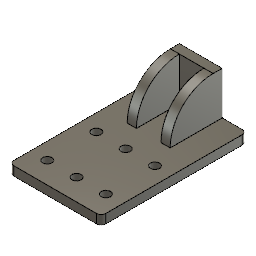
Small_solenoid_basereworkedV1 (Autodesk Fusion 360 design; units mm, degrees)
Autodesk Fusion 360 part; units mm, degrees
note: some values were not read from the file. Set by a fixed rule: which sketch regions a step uses.
sketch "Sketch1" plane through (0, 0, 0) normal (0, 1, 0) x (1, 0, 0)
  line L0 (-15, 15.25) -> (15, 15.25)
  line L1 (15, 15.25) -> (15, -15.25)
  line L2 (15, -15.25) -> (-15, -15.25)
  line L3 (-15, -15.25) -> (-15, 15.25)
  line L4 (-15, 15.25) -> (15, -15.25) construction
  line L5 (15, 15.25) -> (-15, -15.25) construction
  dimension "d1" = 30.5
  dimension "d2" = 30
extrude "Extrude1" add sketch "Sketch1" along normal blind 3
sketch "Sketch2" plane through (0, 0, -15.25) normal (0, 0, -1) x (-1, 0, 0)
  line L0 (-15, 0) -> (15, 0)
  line L1 (15, 0) -> (15, 3)
  line L2 (15, 3) -> (-15, 3)
  line L3 (-15, 3) -> (-15, 0)
  line L4 (7, 0) -> (-7, 0)
  line L5 (-7, 0) -> (-7, 17)
  line L6 (-7, 17) -> (7, 17)
  line L7 (7, 17) -> (7, 0)
  line L8 (7, 1.5) -> (15, 1.5) construction
  line L9 (-15, 1.5) -> (-7, 1.5) construction
  dimension "d5" = 14
  dimension "d6" = 14
  measures "d5" distance of L2 L6
extrude "Extrude2" add sketch "Sketch2" against normal blind 3 contours L2 L5 L6 L7
sketch "Sketch3" plane through (7, 0, 0) normal (1, 0, 0) x (0, 0, -1)
  line L0 (15.25, 3) -> (15.25, 17)
  line L1 (15.25, 17) -> (12.25, 17)
  line L2 (12.25, 17) -> (12.25, 3)
  line L3 (12.25, 3) -> (15.25, 3)
  arc A0 (12.25, 17) -> (-1.75, 3) centre (12.25, 3) ccw
  line L4 (-15.25, 3) -> (15.25, 3)
extrude "Extrude3" add sketch "Sketch3" against normal blind 3 contours L2 A0 L4
sketch "Sketch7" plane through (-7, 0, 0) normal (-1, 0, 0) x (0, 0, 1)
  line L0 (-15.25, 17) -> (-15.25, 3)
  line L1 (-15.25, 3) -> (-12.25, 3)
  line L2 (-12.25, 3) -> (-12.25, 17)
  line L3 (-12.25, 17) -> (-15.25, 17)
  arc A0 (1.75, 3) -> (-12.25, 17) centre (-12.25, 3) ccw
  line L4 (-12.25, 3) -> (1.75, 3)
extrude "Extrude4" add sketch "Sketch7" against normal blind 3 contours L2 A0 L4
sketch "Sketch9" plane through (0, 0, -15.25) normal (0, 0, -1) x (-1, 0, 0)
  line L0 (-15, 0) -> (15, 0)
  line L1 (15, 0) -> (15, 3)
  line L2 (15, 3) -> (7, 3)
  line L3 (7, 3) -> (7, 17)
  line L4 (7, 17) -> (-7, 17)
  line L5 (-7, 17) -> (-7, 3)
  line L6 (-7, 3) -> (-15, 3)
  line L7 (-15, 3) -> (-15, 0)
  circle A0 centre (0, 10) radius 1.5
  line L8 (-7, 17) -> (7, 3) construction
  line L9 (-7, 3) -> (7, 17) construction
  dimension "d14" = 3
  measures "d14" diameter of A0
extrude "Extrude5" cut sketch "Sketch9" against normal up to surface (3 mm away) contours A0
extrude "Extrude8" cut 1 faces at (5, 1, 15.25) along direction (0, 0, -1) up to surface (13.5 mm away)
extrude "Extrude9" add 1 faces at (1.3333, 1, 1.75) along direction (0, 0, 1) blind 30.5
sketch "Sketch13" plane through (0, 3, 0) normal (0, 1, 0) x (-1, 0, 0)
  line L0 (-15, 32.25) -> (-15, -15.25)
  line L1 (-15, -15.25) -> (-7, -15.25)
  line L2 (-7, -15.25) -> (-7, 1.75)
  line L3 (-7, 1.75) -> (-4, 1.75)
  line L4 (-4, 1.75) -> (-4, -12.25)
  line L5 (-4, -12.25) -> (4, -12.25)
  line L6 (4, -12.25) -> (4, 1.75)
  line L7 (4, 1.75) -> (7, 1.75)
  line L8 (7, 1.75) -> (7, -15.25)
  line L9 (7, -15.25) -> (15, -15.25)
  line L10 (15, -15.25) -> (15, 32.25)
  line L11 (15, 32.25) -> (-15, 32.25)
  line L12 (9.55, 32.25) -> (9.55, 25.25) construction
  line L13 (9.55, 25.25) -> (-9.55, 25.25)
  line L14 (-9.55, 25.25) -> (-9.55, 32.25) construction
  line L15 (0, 36) -> (0, -16.5331) construction
  line L16 (9.55, 25.25) -> (9.55, 9.25) construction
  line L17 (9.55, 9.25) -> (-9.55, 9.25) construction
  line L18 (-9.55, 9.25) -> (-9.55, 25.25) construction
  circle A0 centre (9.55, 9.25) radius 1.5
  circle A1 centre (-9.55, 9.25) radius 1.5
  circle A2 centre (-9.55, 25.25) radius 1.5
  circle A3 centre (0, 25.25) radius 1.5
  circle A4 centre (9.55, 25.25) radius 1.5
  circle A5 centre (0, 9.25) radius 1.5
  dimension "d49" = 19.1
  dimension "d50" = 7
  dimension "d51" = 16
  dimension "d52" = 3
  dimension "d53" = 3
  dimension "d54" = 3
  dimension "d55" = 3
  dimension "d56" = 3
  dimension "d57" = 3
  measures "d52" diameter of A0
  measures "d53" diameter of A1
  measures "d54" diameter of A2
  measures "d55" diameter of A3
  measures "d56" diameter of A4
  measures "d57" diameter of A5
extrude "Extrude11" cut sketch "Sketch13" against normal up to surface (3 mm away) contours L13 A3 | L13 A3 | A0 | A1 | A2 | A4 | A5
fillet "Fillet1" radius 1.5 4 edges at (-15, 1.5, 32.25) (15, 1.5, 32.25) (15, 1.5, -15.25) (-15, 1.5, -15.25)
